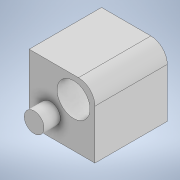
# Autodesk Inventor part: spacer dubbele hoogte behuizing zonder magneet
Saved by Autodesk Inventor 2021 (Build 250183000, 183)
## iProperties
Created: 2023-11-14
Part Number: spacer dubbele hoogte behuizing zonder magneet
Material: Generic
Document SubType Name: Modeling
Designer: Elias
Density: 1 g/cm^3
Appearance: Default
Author: Elias
Autodesk Inventor part; units mm, degrees
ref_plane "YZ Plane" through (0, 0, 0) normal (1, 0, 0) x (0, 1, 0)
ref_plane "XZ Plane" through (0, 0, 0) normal (0, 1, 0) x (-1, 0, 0)
ref_plane "XY Plane" through (0, 0, 0) normal (0, 0, 1) x (1, 0, 0)
sketch "Sketch1" plane through (0, 0, 0) normal (0, 0, 1) x (1, 0, 0)
  line L0 (5, 0) -> (20, 0)
  line L1 (20, 0) -> (20, 15)
  line L2 (15, 20) -> (0, 20)
  line L3 (0, 20) -> (0, 5)
  arc A0 (20, 15) -> (15, 20) centre (15, 15) ccw
  arc A1 (0, 5) -> (5, 0) centre (5, 5) ccw
  point P0 (0, 0)
  point P1 (20, 20)
  dimension "d0" = 20
  dimension "d1" = 20
  dimension "d4" = 5
  dimension "d5" = 5
  constraints: 8 end point, 4 point on circle, 4 point on line, 4 tangent, 2 centre point, 2 parallel, 1 horizontal, 1 perpendicular
  measures "d0" distance of point (20, 20) L2.end
  measures "d1" distance of L0.end point (20, 20)
  measures "d4" radius of A0
  measures "d5" radius of A1
extrude "Extrusion1" add sketch "Sketch1" along normal blind 22
sketch "Sketch2" plane through (0, 0, 22) normal (0, 0, 1) x (1, 0, 0)
  line L0 (15, 20) -> (0, 20) projected
  line L1 (20, 0) -> (20, 15) projected
  point P0 (0, 0)
  point P1 (13.5, 13.5)
  dimension "d13" = 6.5
  dimension "d14" = 6.5
  measures "d13" distance from line of L0 point (13.5, 13.5)
  measures "d14" distance from line of L1 point (13.5, 13.5)
hole "Hole1" at (13.5, 13.5, 22) direction (0, 0, -1) diameter 10 depth 16
sketch "Sketch3" plane through (13.5, 13.5, 6) normal (0, 0, 1) x (1, 0, 0)
  line L0 (6.5, -13.5) -> (6.5, 1.5) projected
  line L1 (1.5, 6.5) -> (-13.5, 6.5) projected
  point P0 (-13.5, -13.5)
  point P1 (0, 0)
  dimension "d22" = 6.5
  dimension "d23" = 6.5
  measures "d22" distance from line of L0 point (0, 0)
  measures "d23" distance from line of L1 point (0, 0)
hole "Hole2" at (13.5, 13.5, 6) direction (0, 0, -1) diameter 3 depth 16
sketch "Sketch4" plane through (0, 0, 22) normal (0, 0, 1) x (1, 0, 0)
  circle A0 centre (6.5, 6.5) radius 3
  line L0 (5, 0) -> (20, 0) projected
  line L1 (0, 20) -> (0, 5) projected
  point P0 (0, 0)
  dimension "d24" = 6
  dimension "d25" = 6.5
  dimension "d26" = 6.5
  constraints: 1 centre point
  measures "d24" diameter of A0
  measures "d25" distance from line of L0 A0.centre
  measures "d26" distance from line of L1 A0.centre
extrude "Extrusion2" add sketch "Sketch4" along normal blind 5
body "Solid1"
